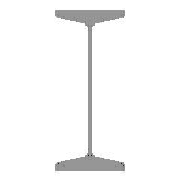
# Autodesk Inventor part: ISO 657/15 - SB 120x12 - 1293
Saved by Autodesk Inventor 2021 (Build 250183000, 183)
## iProperties
_CCFamilyMember: 3
_CCFamilyDisplayName: ISO 657/15 - Профили горячекатаные стальные. Часть 15. Балки двутавровые с наклонными полками (метрическая серия). Размеры и характеристики поперечного сечения
_FrameMemberDoc: Frame Member File
_Version: 15.0.0
_GetPNFromCC: 1
Created: 2020-09-20
Part Number: ISO 657/15 - SB 120x12 - 1293
Material: Сталь, мягкая
Description: Профили горячекатаные стальные. Часть 15. Балки двутавровые с наклонными полками (метрическая серия). Размеры и характеристики поперечного сечения
Document SubType Name: Modeling
Standard: ISO 657/15
Designer: Kostya
Standard Revision: First edition 1980-09-15
Standards Organization: ISO
Language: ru-RU
Size Designation: SB 120x12
Categories: <MemberInstance><Categories><Category DisplayName="Профили фасонные" InternalName="089c4875-fa83-4c05-b084-43b9cc11f5ed" Mnemonic="GRDR"><CategoryParameter DisplayName="Вес погонного метра" InternalName="0bb95a10-148f-4027-a459-38d7b056702a" Mnemonic="shpmass"/><CategoryParameter DisplayName="Площадь сечения" InternalName="1ff91680-64b0-4202-b9a3-7fd3f94bba3b" Mnemonic="secarea"/><CategoryParameter DisplayName="Радиус инерции (x)" InternalName="25778675-03e9-40c1-b6a8-4a9ed693320d" Mnemonic="gyrradx"/><CategoryParameter DisplayName="Модуль жесткости при кручении" InternalName="26c1ec35-5026-4c63-ad0a-751cf684a536" Mnemonic="torrigmod"/><CategoryParameter DisplayName="Расстояние центра тяжести X-X" InternalName="26c9bdb8-9c79-4b4f-a92e-8e197583c9c4" Mnemonic="grcendistX"/><CategoryParameter DisplayName="Старое обозначение элемента" InternalName="340afe4f-75d7-48d3-ab7d-943f3c3da468" Mnemonic="LegacyMemberID"/><CategoryParameter DisplayName="Основная длина" InternalName="42e34263-8f20-4d0e-ad48-bf1385b87c24" Mnemonic="shplen"/><CategoryParameter DisplayName="Момент инерции (y)" InternalName="4b9f58ea-bced-460e-81ea-3d29ca5a49e3" Mnemonic="inermomy"/><CategoryParameter DisplayName="Момент инерции (x)" InternalName="4cd780bc-73d7-43ac-917a-579e5cbd684d" Mnemonic="inermomx"/><CategoryParameter DisplayName="Настраиваемые базовые точки" InternalName="4f1d1b73-316d-484b-a3df-9cbabb16eb77" Mnemonic="shpBasePoint"/><CategoryParameter DisplayName="Высота фигуры" InternalName="50274e7d-5ac0-4796-92cb-c59e54983c67" Mnemonic="shpheig"/><CategoryParameter DisplayName="Момент сопротивления сечения (y)" InternalName="59eaa5e9-d227-48dc-b6c1-6920f96e0f95" Mnemonic="secmody"/><CategoryParameter DisplayName="Обозначение разреза" InternalName="5a64d034-428d-49c8-ba32-7619764de20f" Mnemonic="shpdes"/><CategoryParameter DisplayName="Момент сопротивления сечения (x)" InternalName="72cfad18-cf51-4ed4-aaa7-c6b224f8419f" Mnemonic="secmodx"/><CategoryParameter DisplayName="Торсионный момент сопротивления сечения" InternalName="7c55a8dc-8844-49f9-a867-cc677b30ec9a" Mnemonic="torsecmod"/><CategoryParameter DisplayName="Ширина фигуры" InternalName="7c717d54-a18f-4666-b4d4-573cce22c62c" Mnemonic="shpwdth"/><CategoryParameter DisplayName="Толщина второй фигуры" InternalName="9251a8e1-85fd-4e47-af99-afdb762317d9" Mnemonic="shpthick2"/><CategoryParameter DisplayName="Созданные с помощью генератора рам" InternalName="9c666724-f362-4ea7-ac62-f6a007de5c69" Mnemonic="shpFGAuto"/><CategoryParameter DisplayName="Расстояние центра тяжести Y-Y" InternalName="bcc4fb17-7af4-436a-8f8c-d0aa3b0248c5" Mnemonic="grcendistY"/><CategoryParameter DisplayName="Радиус инерции (y)" InternalName="bfa18ebe-1636-4dbe-8d42-b263e0b73184" Mnemonic="gyrrady"/><CategoryParameter DisplayName="Толщина фигуры" InternalName="d109cf76-8eb4-42fc-9800-4409734adc67" Mnemonic="shpthick"/><CategoryParameter DisplayName="Коэффициент смещения при сдвиге" InternalName="de4c90c6-aaa8-468f-a335-6737b311b5d3" Mnemonic="shdispc"/><Category DisplayName="Двутавры" InternalName="6918ea94-8af8-4304-ae03-7d2c1ce55d4b" Mnemonic="ISHP"><CategoryParameter DisplayName="Вес погонного метра" InternalName="0dc32564-f4aa-4aa4-8c75-62cb498c92c3" Mnemonic="shpmass"/><CategoryParameter DisplayName="Радиус инерции (y)" InternalName="0f8afd8f-b9f7-472e-8e75-9212891574fd" Mnemonic="gyrrady"/><CategoryParameter DisplayName="Толщина второй фигуры" InternalName="391ebf09-f515-4c94-817f-86f5e53f4689" Mnemonic="shpthick2"/><CategoryParameter DisplayName="Момент инерции (x)" InternalName="a758f08a-3b45-4a09-8ee4-ba904e580c14" Mnemonic="inermomx"/><CategoryParameter DisplayName="Момент инерции (y)" InternalName="ae881498-39b5-464d-9622-212b1cfb5926" Mnemonic="inermomy"/><CategoryParameter DisplayName="Площадь сечения" InternalName="bf9dd762-a4b6-4f54-802b-8b144141f7fb" Mnemonic="secarea"/><CategoryParameter DisplayName="Момент сопротивления сечения (y)" InternalName="c0ad6f84-71f4-4f7a-a8c1-bbe4f36d703a" Mnemonic="secmody"/><CategoryParameter DisplayName="Толщина фигуры" InternalName="c729d173-373e-41ba-bff7-d28a079d944c" Mnemonic="shpthick"/><CategoryParameter DisplayName="Радиус инерции (x)" InternalName="db90017b-4fac-4daa-80b0-a7886743939d" Mnemonic="gyrradx"/><CategoryParameter DisplayName="Момент сопротивления сечения (x)" InternalName="e71bf9c5-e82b-494f-914d-abe97254150e" Mnemonic="secmodx"/><CategoryParameter DisplayName="Ширина фигуры" InternalName="f705f81c-b398-4253-aed1-763ae4858594" Mnemonic="shpwdth"/></Category></Category><Category DisplayName="ТипДанных" InternalName="23b78d0f-2648-40c6-8793-ca6db495c9e8" Mnemonic="DATATYPE"><CategoryParameter DisplayName="ОтображаемоеИмя" InternalName="05415f3d-3907-474b-a020-eb9d644f4cf3" Mnemonic="DISPLAYNAME"/><CategoryParameter DisplayName="Стандарт" InternalName="0c0a119c-1e12-4c84-803f-101930972f5e" Mnemonic="STANDARD"/><CategoryParameter DisplayName="Наименование" InternalName="13903e3d-64b1-4950-80da-f627842ea37f" Mnemonic="DESCRIPTION"/><CategoryParameter DisplayName="Обозначение" InternalName="2675968c-4ce5-49e0-a4f5-552d29089031" Mnemonic="DESIGNATION"/><CategoryParameter DisplayName="Строка по умолчанию" InternalName="2af9ec52-faaa-4026-b378-f9fa4afca842" Mnemonic="DEFAULTROW"/><CategoryParameter DisplayName="Имя папки" InternalName="3f06958e-8713-4116-9be7-ed6184ecc97b" Mnemonic="FOLDERNAME"/><CategoryParameter DisplayName="Указатель редакций" InternalName="45a75005-10b1-4dfc-8d6d-dfe629f0b93c" Mnemonic="REVISIONGUID"/><CategoryParameter DisplayName="ИмяФайла" InternalName="8b46a4cc-9585-4fed-90c3-899f57e09a73" Mnemonic="FILENAME"/><CategoryParameter DisplayName="ОргСтанд" InternalName="8f5914e1-4693-403f-8ab5-d37768198c9d" Mnemonic="STDSORG"/><CategoryParameter DisplayName="Версия семейства" InternalName="914462f6-6e19-4b14-ba84-155b9680b1d0" Mnemonic="FAMILYREVISION"/><CategoryParameter DisplayName="Редакция стандарта" InternalName="91d5a463-65c2-4fde-b823-3b7fea5e8e17" Mnemonic="STANDARDREVISION"/><CategoryParameter DisplayName="редакция элемента" InternalName="a65d44b9-392f-4f4f-857b-e4b3d54996fe" Mnemonic="MEMBERREVISION"/><CategoryParameter DisplayName="ФорматКлипа" InternalName="bc51e27b-3422-4e78-93ef-cec197ddf230" Mnemonic="CLIPFORMAT"/><CategoryParameter DisplayName="Изготовитель" InternalName="cd6c7a72-a28a-4e50-99a9-2c7f4e13e5ad" Mnemonic="MANUFACTURER"/><CategoryParameter DisplayName="ВнутреннееИмя" InternalName="cf1d0246-76d9-4b4a-8305-fa0409afb5c1" Mnemonic="INTERNALNAME"/><CategoryParameter DisplayName="Метрическая" InternalName="e2385c5b-1ea4-4823-96a8-8de651266ec3" Mnemonic="ISMETRIC"/><Category DisplayName="Деталь" InternalName="c0e0b642-3bcb-4cc8-9e80-f96d35c4afa4" Mnemonic="PART"><CategoryParameter DisplayName="Номер детали" InternalName="016b6077-bfbe-49bd-92c9-d8d59c39c941" Mnemonic="PARTNUMBER"/><CategoryParameter DisplayName="Инвентарный номер" InternalName="4dba7c1c-e26c-444e-836c-b08b433409a8" Mnemonic="STOCKNUMBER"/><CategoryParameter DisplayName="Ключ материала" InternalName="5c9a8adb-dd2b-4535-b97f-0a94a95fe41f" Mnemonic="MATERIALKEY"/><CategoryParameter DisplayName="Материал" InternalName="818a152a-d3c3-49ca-80ee-df7d91421b8e" Mnemonic="MATERIAL"/></Category></Category><Category DisplayName="СтараяКарта" InternalName="cd87c42b-3e48-431e-b5c0-1cbeb14dfe77" Mnemonic="LEGACYMAP"><CategoryParameter DisplayName="уникальное обозначение элемента DA" InternalName="0918ad47-427f-4fed-ae26-24c81c58f590" Mnemonic="DACOOKIE"/><CategoryParameter DisplayName="Объединить код 11" InternalName="0ee8fb18-e2ed-4f39-96f6-1f4b5f50aa71" Mnemonic="MERGE11"/><CategoryParameter DisplayName="уникальное обозначение элемента CC" InternalName="5193edd4-b2b0-4ab4-9d54-de900eee34e0" Mnemonic="CCCOOKIE"/><CategoryParameter DisplayName="Разделить код" InternalName="72b5c83c-be7f-45c4-ae51-9160ea6deb26" Mnemonic="SPLIT"/><CategoryParameter DisplayName="КодУчастника" InternalName="8e5e0294-fc51-4c8f-b3d7-003dc5ed94f6" Mnemonic="MEMBERID"/><CategoryParameter DisplayName="ИмяКаталога" InternalName="d99d1e27-aa94-4de2-af4c-c348882a6f4f" Mnemonic="CATALOGNAME"/><CategoryParameter DisplayName="НомерСемейства" InternalName="e705e1f4-09cb-413e-91f9-551b4188271e" Mnemonic="FAMILYNUMBER"/></Category></Categories><FamilyTemplate Id="gp0201"><FamilyTemplateParameters><FamilyTemplateParameter ObjectType="kUserParameterObject" ValueType="xs:double" Id="1" ObjectReferenceKey="G_C"/><FamilyTemplateParameter ObjectType="kUserParameterObject" ValueType="xs:double" Id="7" ObjectReferenceKey="B_L"/><FamilyTemplateParameter ObjectType="kUserParameterObject" ValueType="xs:double" Id="8" ObjectReferenceKey="G_IR"/><FamilyTemplateParameter ObjectType="kUserParameterObject" ValueType="xs:double" Id="10" ObjectReferenceKey="G_W"/><FamilyTemplateParameter ObjectType="kUserParameterObject" ValueType="xs:double" Id="11" ObjectReferenceKey="G_T"/><FamilyTemplateParameter ObjectType="kUserParameterObject" ValueType="xs:double" Id="12" ObjectReferenceKey="G_H"/><FamilyTemplateParameter ObjectType="kUserParameterObject" ValueType="xs:double" Id="14" ObjectReferenceKey="G_ER"/><FamilyTemplateParameter ObjectType="kUserParameterObject" ValueType="xs:double" Id="15" ObjectReferenceKey="G_T1"/><FamilyTemplateParameter ObjectType="kUserParameterObject" ValueType="xs:double" Id="16" ObjectReferenceKey="G_NG"/><FamilyTemplateParameter ObjectType="kPropertyObject" ValueType="xs:string" Id="100" ObjectReferenceKey="{32853F0F-3444-11d1-9E93-0060B03C1CA6}" SubObjectId="52"/><FamilyTemplateParameter ObjectType="kPropertyObject" ValueType="xs:string" Id="105" ObjectReferenceKey="{32853F0F-3444-11d1-9E93-0060B03C1CA6}" SubObjectId="5"/><FamilyTemplateParameter ObjectType="kPartComponentDefinitionObject" ValueType="xs:string" Id="110" SubObjectId="Material"/><FamilyTemplateParameter ObjectType="kPropertyObject" ValueType="xs:string" Id="112" ObjectReferenceKey="{32853F0F-3444-11d1-9E93-0060B03C1CA6}" SubObjectId="55"/></FamilyTemplateParameters></FamilyTemplate><CategoryParameterMap><ParamToTemplateMap><ParamToTemplate CategoryParameter="//CategoryParameter[@InternalName='05415f3d-3907-474b-a020-eb9d644f4cf3']" ConstantValue="ISO 657/15"/><ParamToTemplate CategoryParameter="//CategoryParameter[@InternalName='cf1d0246-76d9-4b4a-8305-fa0409afb5c1']" ConstantValue="8a2f1b25-ac0d-44bf-b636-e7398752dea3"/><ParamToTemplate CategoryParameter="//CategoryParameter[@InternalName='3f06958e-8713-4116-9be7-ed6184ecc97b']" ConstantValue="ISO 657 15"/><ParamToTemplate CategoryParameter="//CategoryParameter[@InternalName='914462f6-6e19-4b14-ba84-155b9680b1d0']" ConstantValue="10"/><ParamToTemplate CategoryParameter="//CategoryParameter[@InternalName='bc51e27b-3422-4e78-93ef-cec197ddf230']" ConstantValue="CF_INVENTOR.STDPARTS"/><ParamToTemplate CategoryParameter="//CategoryParameter[@InternalName='e2385c5b-1ea4-4823-96a8-8de651266ec3']" ConstantValue="true"/><ParamToTemplate CategoryParameter="//CategoryParameter[@InternalName='13903e3d-64b1-4950-80da-f627842ea37f']" ConstantValue="Hot-rolled steel sections-part 15: sloping flange  beam sections (metric series) - Dimensions and sectional properties"/><ParamToTemplate CategoryParameter="//CategoryParameter[@InternalName='8f5914e1-4693-403f-8ab5-d37768198c9d']" ConstantValue="ISO"/><ParamToTemplate CategoryParameter="//CategoryParameter[@InternalName='0c0a119c-1e12-4c84-803f-101930972f5e']" ConstantValue="ISO 657/15"/><ParamToTemplate CategoryParameter="//CategoryParameter[@InternalName='cd6c7a72-a28a-4e50-99a9-2c7f4e13e5ad']" TemplateParameter="104"/><ParamToTemplate CategoryParameter="//CategoryParameter[@InternalName='91d5a463-65c2-4fde-b823-3b7fea5e8e17']" ConstantValue="First edition 1980-09-15"/><ParamToTemplate CategoryParameter="//CategoryParameter[@InternalName='45a75005-10b1-4dfc-8d6d-dfe629f0b93c']" ConstantValue="6de6a5fd-1ce5-4d12-b53d-70f4d0e47883"/><ParamToTemplate CategoryParameter="//CategoryParameter[@InternalName='2af9ec52-faaa-4026-b378-f9fa4afca842']" ConstantValue="1"/><ParamToTemplate CategoryParameter="//CategoryParameter[@InternalName='9c666724-f362-4ea7-ac62-f6a007de5c69']" ConstantValue="1"/><ParamToTemplate CategoryParameter="//CategoryParameter[@InternalName='d99d1e27-aa94-4de2-af4c-c348882a6f4f']" ConstantValue="ISO"/><ParamToTemplate CategoryParameter="//CategoryParameter[@InternalName='e705e1f4-09cb-413e-91f9-551b4188271e']" ConstantValue="144"/><ParamToTemplate CategoryParameter="//CategoryParameter[@InternalName='8b46a4cc-9585-4fed-90c3-899f57e09a73']" ConstantValue="ISO 657/15 - SB 120x12 - 0,001"/><ParamToTemplate CategoryParameter="//CategoryParameter[@InternalName='a65d44b9-392f-4f4f-857b-e4b3d54996fe']" ConstantValue="4DAE484A-2C0F-4BF9-A417-EB1810DB03F6"/><ParamToTemplate CategoryParameter="//CategoryParameter[@InternalName='bf9dd762-a4b6-4f54-802b-8b144141f7fb']" ConstantValue="14.7"/><ParamToTemplate CategoryParameter="//CategoryParameter[@InternalName='de4c90c6-aaa8-468f-a335-6737b311b5d3']" ConstantValue="2,45"/><ParamToTemplate CategoryParameter="//CategoryParameter[@InternalName='db90017b-4fac-4daa-80b0-a7886743939d']" ConstantValue="4,83"/><ParamToTemplate CategoryParameter="//CategoryParameter[@InternalName='0f8afd8f-b9f7-472e-8e75-9212891574fd']" ConstantValue="1,27"/><ParamToTemplate CategoryParameter="//CategoryParameter[@InternalName='a758f08a-3b45-4a09-8ee4-ba904e580c14']" ConstantValue="342"/><ParamToTemplate CategoryParameter="//CategoryParameter[@InternalName='ae881498-39b5-464d-9622-212b1cfb5926']" ConstantValue="23,5"/><ParamToTemplate CategoryParameter="//CategoryParameter[@InternalName='e71bf9c5-e82b-494f-914d-abe97254150e']" ConstantValue="57"/><ParamToTemplate CategoryParameter="//CategoryParameter[@InternalName='c0ad6f84-71f4-4f7a-a8c1-bbe4f36d703a']" ConstantValue="7,84"/><ParamToTemplate CategoryParameter="//CategoryParameter[@InternalName='5a64d034-428d-49c8-ba32-7619764de20f']" ConstantValue="SB 120x12"/><ParamToTemplate CategoryParameter="//CategoryParameter[@InternalName='8e5e0294-fc51-4c8f-b3d7-003dc5ed94f6']" ConstantValue="3"/><ParamToTemplate CategoryParameter="//CategoryParameter[@InternalName='42e34263-8f20-4d0e-ad48-bf1385b87c24']" TemplateParameter="7"/><ParamToTemplate CategoryParameter="//CategoryParameter[@InternalName='2675968c-4ce5-49e0-a4f5-552d29089031']" TemplateParameter="100"/><ParamToTemplate CategoryParameter="//CategoryParameter[@InternalName='50274e7d-5ac0-4796-92cb-c59e54983c67']" TemplateParameter="12"/><ParamToTemplate CategoryParameter="//CategoryParameter[@InternalName='818a152a-d3c3-49ca-80ee-df7d91421b8e']" TemplateParameter="110"/><ParamToTemplate CategoryParameter="//CategoryParameter[@InternalName='016b6077-bfbe-49bd-92c9-d8d59c39c941']" TemplateParameter="105"/><ParamToTemplate CategoryParameter="//CategoryParameter[@InternalName='4dba7c1c-e26c-444e-836c-b08b433409a8']" TemplateParameter="112"/></ParamToTemplateMap></CategoryParameterMap></MemberInstance>
Stock Number: SB 120x12
Density: 7.85 g/cm^3
Appearance: С умеренной полировкой
IsCustomPart: 1
G_L: 1293,000 мм
G_W: 60,000 мм
G_H: 120,000 мм
+9AE85581-1BDB-489F-A98D-5D93BF578E77+ВЫНОСНОЙЭЛЕМЕНТ1: Врезать
+DF751051-F2AA-4D9E-8944-BBA44DBFD974+ВЫНОСНОЙЭЛЕМЕНТ2: Врезать
Author: Kostya
Autodesk Inventor part; units mm, degrees
ref_plane "YZ Plane" through (0, 0, 0) normal (1, 0, 0) x (0, 1, 0)
ref_plane "XZ Plane" through (0, 0, 0) normal (0, 1, 0) x (-1, 0, 0)
ref_plane "XY Plane" through (0, 0, 0) normal (0, 0, 1) x (1, 0, 0)
ref_plane "Начальная плоскость" through (0, 0, 0) normal (0, 0, 1) x (1, 0, 0)
ref_plane "Конечная плоскость" through (0, 0, 1300) normal (0, 0, 1) x (1, 0, 0)
sketch "Эскиз" plane through (0, 0, 0) normal (0, 0, 1) x (1, 0, 0)
  line L0 (-2.5, 0) -> (-2.5, -43.5133)
  line L1 (-9.3866, -51.4354) -> (-26.5567, -53.8485)
  line L2 (-30, -57.8096) -> (-30, -60)
  line L3 (-30, -60) -> (0, -60)
  line L4 (-16.25, -60) -> (-16.25, -52.4) construction
  line L5 (-25.7112, 0) -> (34.2816, 0) construction
  line L6 (0, 40) -> (0, -60) construction
  line L7 (0, -48) -> (0, 64) construction
  line L8 (2.5, 0) -> (2.5, -43.5133)
  line L9 (9.3866, -51.4354) -> (26.5567, -53.8485)
  line L10 (30, -57.8096) -> (30, -60)
  line L11 (30, -60) -> (0, -60)
  line L12 (-2.5, 0) -> (2.5, 0) construction
  line L13 (-2.5, 0) -> (-2.5, 43.5133)
  line L14 (-9.3866, 51.4354) -> (-26.5567, 53.8485)
  line L15 (-30, 57.8096) -> (-30, 60)
  line L16 (-30, 60) -> (0, 60)
  line L17 (2.5, 0) -> (2.5, 43.5133)
  line L18 (9.3866, 51.4354) -> (26.5567, 53.8485)
  line L19 (30, 57.8096) -> (30, 60)
  line L20 (30, 60) -> (0, 60)
  arc A0 (-30, 57.8096) -> (-26.5567, 53.8485) centre (-26, 57.8096) ccw
  arc A1 (26.5567, 53.8485) -> (30, 57.8096) centre (26, 57.8096) ccw
  arc A2 (30, -57.8096) -> (26.5567, -53.8485) centre (26, -57.8096) ccw
  arc A3 (-26.5567, -53.8485) -> (-30, -57.8096) centre (-26, -57.8096) ccw
  arc A4 (-2.5, 43.5133) -> (-9.3866, 51.4354) centre (-10.5, 43.5133) ccw
  arc A5 (9.3866, 51.4354) -> (2.5, 43.5133) centre (10.5, 43.5133) ccw
  arc A6 (2.5, -43.5133) -> (9.3866, -51.4354) centre (10.5, -43.5133) ccw
  arc A7 (-9.3866, -51.4354) -> (-2.5, -43.5133) centre (-10.5, -43.5133) ccw
  line L21 (0, 88.8) -> (0, -84.8) construction
  line L22 (-43.7449, 0) -> (47.286, 0) construction
  point P0 (-2.5, -50.4676)
  point P1 (-30, -54.3324)
  point P2 (2.5, -50.4676)
  point P3 (30, -54.3324)
  point P4 (16.25, -60)
  point P5 (16.25, -52.4)
  point P6 (-2.5, 50.4676)
  point P7 (-30, 54.3324)
  point P8 (-16.25, 60)
  point P9 (-16.25, 52.4)
  point P10 (2.5, 50.4676)
  point P11 (30, 54.3324)
  point P12 (16.25, 52.4)
  point P13 (16.25, 60)
  dimension "d1" = 1.9324
  dimension "d2" = 7.6
  dimension "d3" = 13.75
  dimension "d4" = 2.5
  dimension "d5" = 30
  dimension "d10" = 60
  dimension "d14" = 4
  dimension "d15" = 8
  constraints: 42 end point, 24 point on line, 17 symmetric about line, 16 point on circle, 16 tangent, 8 centre point, 6 equal radius, 4 collinear, 1 parallel, 1 perpendicular, 12 other
  measures "d1" vertical distance of point (-30, -54.332) L4.end
  measures "d2" vertical distance of L2.end L4.end
  measures "d3" distance between parallel lines of L4 L2
  measures "d4" distance between parallel lines of L0 L6
  measures "d5" distance between parallel lines of L6 L2
  measures "d10" distance from line of L0.start L3
  measures "d14" radius of A0
  measures "d15" radius of A4
extrude "Тело" add sketch "Эскиз" along normal up to surface (1300 mm away) from surface at 0
sketch "Sketch3" plane through (0, 0, 0) normal (0, 0, 1) x (1, 0, 0)
  line L0 (0, 0) -> (10, 0)
ref_plane "Work Plane3" through (0, 0, 0) normal (0, -1, 0) x (1, 0, 0)
sketch "Sketch4" plane through (0, 0, 0) normal (0, -1, 0) x (1, 0, 0)
  line L0 (-2, 0) -> (12, 0)
  line L1 (-2, 1300) -> (12, 1300)
  dimension "d19" = 1300
  measures "d19" distance between parallel lines of L0 L1
ref_plane "РабПлоскость4" through (784.5, 0, -70) normal (0.7071068, 0, 0.7071068) x (0.7071068, 0, -0.7071068)
ref_plane "РабПлоскость5" through (-2210.5, 0, -70) normal (-0.7071068, 0, 0.7071068) x (0.7071068, 0, 0.7071068)
ref_plane "РабПлоскость6" through (-713, 0, 0) normal (-1, 0, 0) x (0, 0, 1)
sketch "Эскиз5" plane through (-713, 0, 0) normal (-1, 0, 0) x (0, 0, 1)
  line L0 (-3.5, 0) -> (-3.5, -42.8956)
  arc A0 (-13.8299, -54.7788) -> (-3.5, -42.8956) centre (-15.5, -42.8956) ccw
  line L1 (-13.8299, -54.7788) -> (-64.835, -61.9471)
  arc A1 (-64.835, -61.9471) -> (-70, -67.8887) centre (-64, -67.8887) ccw
  line L2 (-70, -67.8887) -> (-70, -70)
  line L3 (-70, -70) -> (0, -70)
  line L4 (70, -70) -> (0, -70)
  line L5 (70, -67.8887) -> (70, -70)
  arc A2 (70, -67.8887) -> (64.835, -61.9471) centre (64, -67.8887) ccw
  line L6 (13.8299, -54.7788) -> (64.835, -61.9471)
  arc A3 (3.5, -42.8956) -> (13.8299, -54.7788) centre (15.5, -42.8956) ccw
  line L7 (3.5, 0) -> (3.5, -42.8956)
  line L8 (3.5, 0) -> (3.5, 42.8956)
  arc A4 (13.8299, 54.7788) -> (3.5, 42.8956) centre (15.5, 42.8956) ccw
  line L9 (13.8299, 54.7788) -> (64.835, 61.9471)
  arc A5 (64.835, 61.9471) -> (70, 67.8887) centre (64, 67.8887) ccw
  line L10 (70, 67.8887) -> (70, 70)
  line L11 (70, 70) -> (0, 70)
  line L12 (-70, 70) -> (0, 70)
  line L13 (-70, 67.8887) -> (-70, 70)
  arc A6 (-70, 67.8887) -> (-64.835, 61.9471) centre (-64, 67.8887) ccw
  line L14 (-13.8299, 54.7788) -> (-64.835, 61.9471)
  arc A7 (-3.5, 42.8956) -> (-13.8299, 54.7788) centre (-15.5, 42.8956) ccw
  line L15 (-3.5, 0) -> (-3.5, 42.8956)
  constraints: 32 end point, 16 point on circle, 8 centre point
extrude "Выдавливание2" add sketch "Эскиз5" along normal up to surface separate body starts on plane at (784.5, 0, -70) facing (0.7071068, 0, 0.7071068) surface through (-2210.5, 0, -70) normal (-0.7071068, 0, 0.7071068)
combine bodies "Комбинировать1" operation type subtract main body 1 bodies to subtract 2
ref_plane "РабПлоскость7" through (-2210.5, 0, 1370) normal (-0.7071068, 0, -0.7071068) x (-0.7071068, 0, 0.7071068)
ref_plane "РабПлоскость8" through (784.5, 0, 1370) normal (0.7071068, 0, -0.7071068) x (-0.7071068, 0, -0.7071068)
ref_plane "РабПлоскость9" through (-713, 0, 1300) normal (1, 0, 0) x (0, 0, -1)
sketch "Эскиз6" plane through (-713, 0, 1300) normal (1, 0, 0) x (0, 0, -1)
  line L0 (-3.5, 0) -> (-3.5, -42.8956)
  arc A0 (-13.8299, -54.7788) -> (-3.5, -42.8956) centre (-15.5, -42.8956) ccw
  line L1 (-13.8299, -54.7788) -> (-64.835, -61.9471)
  arc A1 (-64.835, -61.9471) -> (-70, -67.8887) centre (-64, -67.8887) ccw
  line L2 (-70, -67.8887) -> (-70, -70)
  line L3 (-70, -70) -> (0, -70)
  line L4 (70, -70) -> (0, -70)
  line L5 (70, -67.8887) -> (70, -70)
  arc A2 (70, -67.8887) -> (64.835, -61.9471) centre (64, -67.8887) ccw
  line L6 (13.8299, -54.7788) -> (64.835, -61.9471)
  arc A3 (3.5, -42.8956) -> (13.8299, -54.7788) centre (15.5, -42.8956) ccw
  line L7 (3.5, 0) -> (3.5, -42.8956)
  line L8 (3.5, 0) -> (3.5, 42.8956)
  arc A4 (13.8299, 54.7788) -> (3.5, 42.8956) centre (15.5, 42.8956) ccw
  line L9 (13.8299, 54.7788) -> (64.835, 61.9471)
  arc A5 (64.835, 61.9471) -> (70, 67.8887) centre (64, 67.8887) ccw
  line L10 (70, 67.8887) -> (70, 70)
  line L11 (70, 70) -> (0, 70)
  line L12 (-70, 70) -> (0, 70)
  line L13 (-70, 67.8887) -> (-70, 70)
  arc A6 (-70, 67.8887) -> (-64.835, 61.9471) centre (-64, 67.8887) ccw
  line L14 (-13.8299, 54.7788) -> (-64.835, 61.9471)
  arc A7 (-3.5, 42.8956) -> (-13.8299, 54.7788) centre (-15.5, 42.8956) ccw
  line L15 (-3.5, 0) -> (-3.5, 42.8956)
  constraints: 32 end point, 16 point on circle, 8 centre point
extrude "Выдавливание3" add sketch "Эскиз6" along normal up to surface separate body starts on plane at (-2210.5, 0, 1370) facing (-0.7071068, 0, -0.7071068) surface through (784.5, 0, 1370) normal (0.7071068, 0, -0.7071068)
combine bodies "Комбинировать2" operation type subtract main body 1 bodies to subtract 3
equation "\"d2\" = G_T1"
equation "\"d3\" = G_C"
equation "\"d4\" = 0.5 * G_T"
equation "\"d5\" = 0.5 * G_W"
equation "\"d10\" = 0.5 * G_H"
equation "\"d14\" = G_ER"
equation "\"d15\" = G_IR"
equation "\"d6\" = G_L"
equation "\"G_T\" = 5"
equation "\"G_T1\" = 7.6"
equation "\"G_C\" = 13.75"
equation "\"G_NG\" = 0.140541"
equation "\"G_L\" = 1293"
equation "\"G_ER\" = 0.5 * G_IR"
equation "\"G_IR\" = 8"
equation "\"G_OFFSET_START\" = 0"
equation "\"G_OFFSET_END\" = 0"
equation "\"G_W\" = 60"
equation "\"G_H\" = 120"
body "Solid1"
